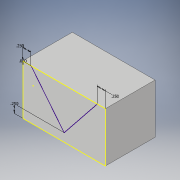
# Autodesk Inventor part: Part2
Saved by Autodesk Inventor 2018 (Build 220112000, 112)
## iProperties
Created: 2018-01-04
Part Number: Part2
Material: Generic
Document SubType Name: Modeling
Designer: 232963
Density: 1 g/cm^3
Appearance: Default
Author: 232963
Autodesk Inventor part; units mm, degrees
ref_plane "YZ Plane" through (0, 0, 0) normal (1, 0, 0) x (0, 1, 0)
ref_plane "XZ Plane" through (0, 0, 0) normal (0, 1, 0) x (-1, 0, 0)
ref_plane "XY Plane" through (0, 0, 0) normal (0, 0, 1) x (1, 0, 0)
sketch "Sketch1" plane through (0, 0, 0) normal (0, 0, 1) x (1, 0, 0)
  line L0 (-8.1507, 12.368) -> (55.3493, 12.368)
  line L1 (55.3493, 12.368) -> (55.3493, -25.732)
  line L2 (55.3493, -25.732) -> (-8.1507, -25.732)
  line L3 (-8.1507, -25.732) -> (-8.1507, 12.368)
  point P0 (0, 0)
  dimension "d0" = 63.5
  dimension "d1" = 38.1
  constraints: 8 end point, 2 parallel, 1 horizontal, 1 perpendicular
  measures "d0" distance of L1.end L2.end
  measures "d1" distance of L0.end L1.end
extrude "Extrusion1" add sketch "Sketch1" along normal blind 38.1
sketch "Sketch2" plane through (0, 0, 38.1) normal (0, 0, 1) x (1, 0, 0)
  line L0 (-1.8007, 12.368) -> (23.5993, -19.382)
  line L1 (23.5993, -19.382) -> (48.9993, 12.368)
  line L2 (55.3493, 12.368) -> (-8.1507, 12.368) projected
  line L3 (-8.1507, 12.368) -> (-8.1507, -25.732) projected
  line L4 (55.3493, -25.732) -> (55.3493, 12.368) projected
  line L5 (-8.1507, -25.732) -> (55.3493, -25.732) projected
  point P0 (0, 0)
  dimension "d4" = 6.35
  dimension "d5" = 0
  dimension "d6" = 6.35
  dimension "d7" = 6.35
  constraints: 4 end point, 1 equal length, 1 point on line
  measures "d4" distance from line of L3 L0.start
  measures "d5" distance from line of L2 L0.start
  measures "d6" distance from line of L4 L1.end
  measures "d7" distance from line of L0.end L5
body "Solid1"
